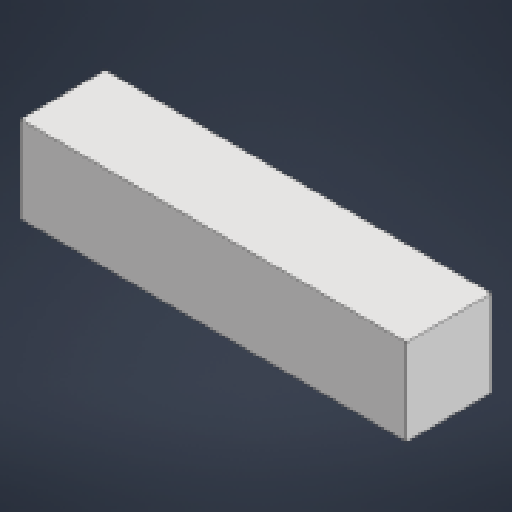
# Autodesk Inventor part: key_v2
Saved by Autodesk Inventor 2026.1 (Build 301233020, 233B)
## iProperties
Created: 2025-11-30
Part Number: key_v2
Material: 일반
Document SubType Name: Modeling
Designer: jaewook
Density: 1 g/cm^3
Appearance: 기본값
Author: jaewook
Autodesk Inventor part; units mm, degrees
ref_plane "YZ Plane" through (0, 0, 0) normal (1, 0, 0) x (0, 1, 0)
ref_plane "XZ Plane" through (0, 0, 0) normal (0, 1, 0) x (-1, 0, 0)
ref_plane "XY Plane" through (0, 0, 0) normal (0, 0, 1) x (1, 0, 0)
sketch "스케치1" plane through (0, 0, 0) normal (1, 0, 0) x (0, 1, 0)
  line L0 (-1.675, 1.65) -> (1.675, 1.65)
  line L1 (1.675, 1.65) -> (1.675, -1.65)
  line L2 (1.675, -1.65) -> (-1.675, -1.65)
  line L3 (-1.675, -1.65) -> (-1.675, 1.65)
  line L4 (-1.675, 1.65) -> (1.675, -1.65) construction
  line L5 (1.675, 1.65) -> (-1.675, -1.65) construction
  point P0 (0, 0)
  dimension "d0" = 3.35
  dimension "d1" = 3.3
  constraints: 12 end point, 2 midpoint, 2 parallel, 1 horizontal, 1 perpendicular
  measures "d0" distance of L1.end L2.end
  measures "d1" distance of L0.end L1.end
extrude "돌출1" add sketch "스케치1" along normal blind 15
